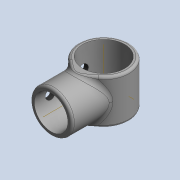
# Autodesk Inventor part: 10-65
Saved by Autodesk Inventor 2021 (Build 250183000, 183)
## iProperties
Created: 2020-04-23
Part Number: 10-65
Material: Generic
Document SubType Name: Modeling
Designer: Hannah
Density: 11.3515 g/cm^3
Appearance: Default
Mass: 250 g
Surface Area: 136.112 cm^2
Volume: 22.0235 cm^3
Author: Hannah
Autodesk Inventor part; units mm, degrees
ref_plane "XY Plane" through (0, 0, 0) normal (0, 0, 1) x (1, 0, 0)
sketch "Sketch1" plane through (0, 0, 0) normal (0, 0, 1) x (1, 0, 0)
  circle A0 centre (0, 0) radius 14
  circle A1 centre (0, 0) radius 17.5
  dimension "d1" = 35
  dimension "d2" = 28
  constraints: 2 centre point, 2 coincident
  measures "d1" diameter of A1
  measures "d2" diameter of A0
extrude "Extrusion1" add sketch "Sketch1" along normal blind 44 contours A0 | A1
sketch "Sketch2" plane through (0, 0, 0) normal (0, 1, 0) x (-1, 0, 0)
  circle A0 centre (0, 0) radius 17.5
  circle A1 centre (0, 0) radius 21
  dimension "d5" = 35
  dimension "d6" = 42
  constraints: 2 centre point, 2 coincident
  measures "d5" diameter of A0
  measures "d6" diameter of A1
extrude "Extrusion2" add sketch "Sketch2" along normal mid plane 37 contours A0 | A1
extrude "Extrusion3" cut sketch "Sketch2" against normal up to surface (37 mm away) from surface at 18.5 contours A0
extrude "Extrusion4" cut sketch "Sketch1" along normal up to surface (44 mm away) contours A0
fillet "Fillet1" radius 5 2 edges at (0.0004, 17.5, 21) (-0.0004, -17.5, 21)
hole "Hole1" at (0, 0, 0) direction (-1, 0, 0) diameter 8.376 end through all thread size "M10x1.5" class "6H" standard "ISO Metric profile"
ref_plane "Work Plane1" through (0, 0, 30.75) normal (0, 0, 1) x (1, 0, 0)
hole "Hole2" at (0, 0, 30.75) direction (-1, 0, 0) diameter 8.376 end through all thread size "M10x1.5" class "6H" standard "ISO Metric profile"
fillet "Fillet2" radius 2 3 edges at (0, 18.5, -21) (-17.5, 0, 44) (0, -18.5, -21)
equation "\"d23\" = -0.5 * d3 + 0.25 * d1"
equation "\"d3\" = 44"
body "Solid1"
